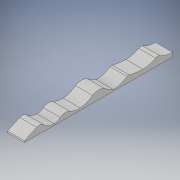
# Autodesk Inventor part: landscape for mars rover
Saved by Autodesk Inventor 2017 (Build 210142000, 142)
## iProperties
Created: 2017-09-12
Part Number: landscape for mars rover
Material: Generic
Document SubType Name: Modeling
Designer: 602199
Density: 1 g/cm^3
Appearance: Default
Author: 602199
Autodesk Inventor part; units mm, degrees
ref_plane "YZ Plane" through (0, 0, 0) normal (1, 0, 0) x (0, 1, 0)
ref_plane "XZ Plane" through (0, 0, 0) normal (0, 1, 0) x (-1, 0, 0)
ref_plane "XY Plane" through (0, 0, 0) normal (0, 0, 1) x (1, 0, 0)
sketch "Sketch1" plane through (0, 0, 0) normal (0, 1, 0) x (-1, 0, 0)
  line L0 (139.7, 1219.2) -> (-139.7, 1219.2)
  line L1 (-139.7, 1219.2) -> (-139.7, -1219.2)
  line L2 (-139.7, -1219.2) -> (139.7, -1219.2)
  line L3 (139.7, -1219.2) -> (139.7, 1219.2)
  line L4 (139.7, 1219.2) -> (-139.7, -1219.2) construction
  line L5 (-139.7, 1219.2) -> (139.7, -1219.2) construction
  point P0 (0, 0)
  dimension "d0" = 279.4
  dimension "d1" = 2438.4
  constraints: 12 end point, 2 midpoint, 2 parallel, 1 horizontal, 1 perpendicular
  measures "d0" distance of L2.end L1.end
  measures "d1" distance of L1.end L0.end
extrude "Extrusion1" add sketch "Sketch1" along normal blind 139.7
sketch "Sketch3" plane through (-139.7, 0, -1219.2) normal (-1, 0, 0) x (0, 0, 1)
  line L0 (2438.4, 139.7) -> (0, 139.7) construction
  line L1 (1219.2, 139.7) -> (1219.2, 0) construction
  line L2 (1219.2, 0) -> (1219.2, 25.4) construction
  line L3 (1219.2, 25.4) -> (0, 25.4)
  line L4 (1219.2, 25.4) -> (2438.4, 25.4)
  line L5 (2438.4, 0) -> (0, 0) construction
  ellipse E0 centre (1219.2024, 69.8468) end of major axis (1342.5189, 69.8468) minor radius 69.85 (1317.8532, 111.7586) -> (1120.5517, 111.7586) ccw
  line L6 (1219.2024, 69.8468) -> (1219.2024, 176.8167) construction
  line L7 (0, 69.85) -> (0, 127.0895)
  line L8 (2438.4, 127.0895) -> (2438.4, 57.2395)
  arc A0 (750.1497, 98.2079) -> (717.7137, 104.389) centre (727.3807, 66.9219) ccw
  arc A1 (0, 69.85) -> (208.3969, 123.3364) centre (0, 502.5771) ccw
  arc A2 (276.8498, 123.3364) -> (208.3969, 123.3364) centre (242.6233, 69.85) ccw
  arc A3 (487.68, 69.85) -> (717.7137, 104.389) centre (471.9739, 957.7485) ccw
  line L9 (135.5865, 91.6403) -> (352.0961, 91.6403) construction
  arc A4 (276.8498, 123.3364) -> (487.68, 69.85) centre (491.8688, 528.6244) ccw
  line L10 (1763.8663, 33.8803) -> (1763.8663, 113.409) construction
  ellipse E1 centre (1763.8663, 33.8803) end of major axis (1865.4663, 33.8803) minor radius 57.271 (1850.0792, 64.183) -> (1693.5763, 75.2333) ccw
  arc A5 (1520.0263, 33.8803) -> (1693.5763, 75.2333) centre (1529.4777, 379.0674) ccw
  arc A6 (975.36, 25.4) -> (1120.5517, 111.7586) centre (657.8319, 724.4807) ccw
  arc A7 (750.1497, 98.2079) -> (975.36, 25.4) centre (973.9324, 405.6999) ccw
  arc A8 (1317.8532, 111.7586) -> (1520.0263, 33.8803) centre (1554.8027, 425.5214) ccw
  arc A9 (2236.968, 117.8247) -> (2124.6268, 99.2248) centre (2194.56, 25.4) ccw
  arc A10 (1850.0792, 64.183) -> (1950.8132, 25.4) centre (1950.8132, 175.6133) ccw
  arc A11 (1950.8132, 25.4) -> (2124.6268, 99.2248) centre (1938.6597, 295.5405) ccw
  line L11 (2236.968, 117.8247) -> (2438.4, 25.4)
  line L12 (2438.4, 57.2395) -> (2438.4, 25.4)
  line L13 (1219.2, 127.0895) -> (1219.2024, 127.0895)
  line L14 (1219.2, 127.0895) -> (1219.2024, 127.0895)
  line L15 (1219.2, 127.0895) -> (1219.2024, 127.0895)
  line L16 (2438.4, 0) -> (2438.4, 139.7) projected
  line L17 (2438.4, 127.0895) -> (2438.4, 139.7)
  line L18 (2438.4, 139.7) -> (0, 139.7)
  line L19 (0, 0) -> (0, 139.7) projected
  line L20 (0, 127.0895) -> (0, 139.7)
  point P0 (729.1332, 155.8475)
  point P1 (243.84, 164.183)
  point P2 (1494.3481, 127.0895)
  dimension "d24" = 101.6
  dimension "d16" = 25.4
  dimension "d23" = 216.5096
  constraints: 34 end point, 26 point on circle, 12 centre point, 6 point on line, 4 collinear, 4 tangent, 3 vertical, 1 coincident, 1 horizontal, 1 midpoint, 1 parallel, 1 perpendicular, 1 symmetric about line, 12 other
  measures "d16" distance of L1.end L2.end
  measures "d23" distance of L9.start L9.end
extrude "Extrusion2" cut sketch "Sketch3" against normal through all contours A7 A0 A3 A4 A2 A1 L7 L19 L18 L16 L8 L12 L11 A9 A11 A10 E1 A5 A8 E0 A6
body "Solid1"
